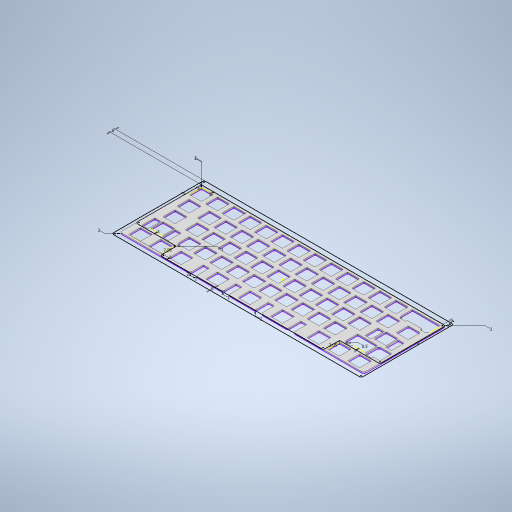
# Autodesk Inventor part: cast
Saved by Autodesk Inventor 2023 (Build 270158000, 158)
## iProperties
Created: 2023-09-13
Part Number: cast
Material: Generic
Document SubType Name: Modeling
Designer: Eric
Density: 1 g/cm^3
Appearance: Default
Author: Eric
Autodesk Inventor part; units mm, degrees
ref_plane "YZ Plane" through (0, 0, 0) normal (1, 0, 0) x (0, 1, 0)
ref_plane "XZ Plane" through (0, 0, 0) normal (0, 1, 0) x (-1, 0, 0)
ref_plane "XY Plane" through (0, 0, 0) normal (0, 0, 1) x (1, 0, 0)
sketch "Sketch1" plane through (0, 0, 0) normal (0, 1, 0) x (-1, 0, 0)
  line L0 (139.85, -45.1) -> (126.85, -45.1)
  line L1 (139.85, -31.1) -> (126.85, -31.1)
  line L2 (140.35, -44.6) -> (140.35, -31.6)
  line L3 (126.35, -44.6) -> (126.35, -31.6)
  arc A0 (139.85, -45.1) -> (140.35, -44.6) centre (139.85, -44.6) ccw
  arc A1 (126.35, -44.6) -> (126.85, -45.1) centre (126.85, -44.6) ccw
  arc A2 (140.35, -31.6) -> (139.85, -31.1) centre (139.85, -31.6) ccw
  arc A3 (126.85, -31.1) -> (126.35, -31.6) centre (126.85, -31.6) ccw
  line L4 (120.8, -45.1) -> (107.8, -45.1)
  line L5 (120.8, -31.1) -> (107.8, -31.1)
  line L6 (121.3, -44.6) -> (121.3, -31.6)
  line L7 (107.3, -44.6) -> (107.3, -31.6)
  arc A4 (120.8, -45.1) -> (121.3, -44.6) centre (120.8, -44.6) ccw
  arc A5 (107.3, -44.6) -> (107.8, -45.1) centre (107.8, -44.6) ccw
  arc A6 (121.3, -31.6) -> (120.8, -31.1) centre (120.8, -31.6) ccw
  arc A7 (107.8, -31.1) -> (107.3, -31.6) centre (107.8, -31.6) ccw
  line L8 (101.75, -45.1) -> (88.75, -45.1)
  line L9 (101.75, -31.1) -> (88.75, -31.1)
  line L10 (102.25, -44.6) -> (102.25, -31.6)
  line L11 (88.25, -44.6) -> (88.25, -31.6)
  arc A8 (101.75, -45.1) -> (102.25, -44.6) centre (101.75, -44.6) ccw
  arc A9 (88.25, -44.6) -> (88.75, -45.1) centre (88.75, -44.6) ccw
  arc A10 (102.25, -31.6) -> (101.75, -31.1) centre (101.75, -31.6) ccw
  arc A11 (88.75, -31.1) -> (88.25, -31.6) centre (88.75, -31.6) ccw
  line L12 (82.7, -45.1) -> (69.7, -45.1)
  line L13 (82.7, -31.1) -> (69.7, -31.1)
  line L14 (83.2, -44.6) -> (83.2, -31.6)
  line L15 (69.2, -44.6) -> (69.2, -31.6)
  arc A12 (82.7, -45.1) -> (83.2, -44.6) centre (82.7, -44.6) ccw
  arc A13 (69.2, -44.6) -> (69.7, -45.1) centre (69.7, -44.6) ccw
  arc A14 (83.2, -31.6) -> (82.7, -31.1) centre (82.7, -31.6) ccw
  arc A15 (69.7, -31.1) -> (69.2, -31.6) centre (69.7, -31.6) ccw
  line L16 (63.65, -45.1) -> (50.65, -45.1)
  line L17 (63.65, -31.1) -> (50.65, -31.1)
  line L18 (64.15, -44.6) -> (64.15, -31.6)
  line L19 (50.15, -44.6) -> (50.15, -31.6)
  arc A16 (63.65, -45.1) -> (64.15, -44.6) centre (63.65, -44.6) ccw
  arc A17 (50.15, -44.6) -> (50.65, -45.1) centre (50.65, -44.6) ccw
  arc A18 (64.15, -31.6) -> (63.65, -31.1) centre (63.65, -31.6) ccw
  arc A19 (50.65, -31.1) -> (50.15, -31.6) centre (50.65, -31.6) ccw
  line L20 (44.6, -45.1) -> (31.6, -45.1)
  line L21 (44.6, -31.1) -> (31.6, -31.1)
  line L22 (45.1, -44.6) -> (45.1, -31.6)
  line L23 (31.1, -44.6) -> (31.1, -31.6)
  arc A20 (44.6, -45.1) -> (45.1, -44.6) centre (44.6, -44.6) ccw
  arc A21 (31.1, -44.6) -> (31.6, -45.1) centre (31.6, -44.6) ccw
  arc A22 (45.1, -31.6) -> (44.6, -31.1) centre (44.6, -31.6) ccw
  arc A23 (31.6, -31.1) -> (31.1, -31.6) centre (31.6, -31.6) ccw
  line L24 (25.55, -45.1) -> (12.55, -45.1)
  line L25 (25.55, -31.1) -> (12.55, -31.1)
  line L26 (26.05, -44.6) -> (26.05, -31.6)
  line L27 (12.05, -44.6) -> (12.05, -31.6)
  arc A24 (25.55, -45.1) -> (26.05, -44.6) centre (25.55, -44.6) ccw
  arc A25 (12.05, -44.6) -> (12.55, -45.1) centre (12.55, -44.6) ccw
  arc A26 (26.05, -31.6) -> (25.55, -31.1) centre (25.55, -31.6) ccw
  arc A27 (12.55, -31.1) -> (12.05, -31.6) centre (12.55, -31.6) ccw
  line L28 (6.5, -45.1) -> (-6.5, -45.1)
  line L29 (6.5, -31.1) -> (-6.5, -31.1)
  line L30 (7, -44.6) -> (7, -31.6)
  line L31 (-7, -44.6) -> (-7, -31.6)
  arc A28 (6.5, -45.1) -> (7, -44.6) centre (6.5, -44.6) ccw
  arc A29 (-7, -44.6) -> (-6.5, -45.1) centre (-6.5, -44.6) ccw
  arc A30 (7, -31.6) -> (6.5, -31.1) centre (6.5, -31.6) ccw
  arc A31 (-6.5, -31.1) -> (-7, -31.6) centre (-6.5, -31.6) ccw
  line L32 (-12.55, -45.1) -> (-25.55, -45.1)
  line L33 (-12.55, -31.1) -> (-25.55, -31.1)
  line L34 (-12.05, -44.6) -> (-12.05, -31.6)
  line L35 (-26.05, -44.6) -> (-26.05, -31.6)
  arc A32 (-12.55, -45.1) -> (-12.05, -44.6) centre (-12.55, -44.6) ccw
  arc A33 (-26.05, -44.6) -> (-25.55, -45.1) centre (-25.55, -44.6) ccw
  arc A34 (-12.05, -31.6) -> (-12.55, -31.1) centre (-12.55, -31.6) ccw
  arc A35 (-25.55, -31.1) -> (-26.05, -31.6) centre (-25.55, -31.6) ccw
  line L36 (-31.6, -45.1) -> (-44.6, -45.1)
  line L37 (-31.6, -31.1) -> (-44.6, -31.1)
  line L38 (-31.1, -44.6) -> (-31.1, -31.6)
  line L39 (-45.1, -44.6) -> (-45.1, -31.6)
  arc A36 (-31.6, -45.1) -> (-31.1, -44.6) centre (-31.6, -44.6) ccw
  arc A37 (-45.1, -44.6) -> (-44.6, -45.1) centre (-44.6, -44.6) ccw
  arc A38 (-31.1, -31.6) -> (-31.6, -31.1) centre (-31.6, -31.6) ccw
  arc A39 (-44.6, -31.1) -> (-45.1, -31.6) centre (-44.6, -31.6) ccw
  line L40 (-50.65, -45.1) -> (-63.65, -45.1)
  line L41 (-50.65, -31.1) -> (-63.65, -31.1)
  line L42 (-50.15, -44.6) -> (-50.15, -31.6)
  line L43 (-64.15, -44.6) -> (-64.15, -31.6)
  arc A40 (-50.65, -45.1) -> (-50.15, -44.6) centre (-50.65, -44.6) ccw
  arc A41 (-64.15, -44.6) -> (-63.65, -45.1) centre (-63.65, -44.6) ccw
  arc A42 (-50.15, -31.6) -> (-50.65, -31.1) centre (-50.65, -31.6) ccw
  arc A43 (-63.65, -31.1) -> (-64.15, -31.6) centre (-63.65, -31.6) ccw
  line L44 (-69.7, -45.1) -> (-82.7, -45.1)
  line L45 (-69.7, -31.1) -> (-82.7, -31.1)
  line L46 (-69.2, -44.6) -> (-69.2, -31.6)
  line L47 (-83.2, -44.6) -> (-83.2, -31.6)
  arc A44 (-69.7, -45.1) -> (-69.2, -44.6) centre (-69.7, -44.6) ccw
  arc A45 (-83.2, -44.6) -> (-82.7, -45.1) centre (-82.7, -44.6) ccw
  arc A46 (-69.2, -31.6) -> (-69.7, -31.1) centre (-69.7, -31.6) ccw
  arc A47 (-82.7, -31.1) -> (-83.2, -31.6) centre (-82.7, -31.6) ccw
  line L48 (-88.75, -45.1) -> (-101.75, -45.1)
  line L49 (-88.75, -31.1) -> (-101.75, -31.1)
  line L50 (-88.25, -44.6) -> (-88.25, -31.6)
  line L51 (-102.25, -44.6) -> (-102.25, -31.6)
  arc A48 (-88.75, -45.1) -> (-88.25, -44.6) centre (-88.75, -44.6) ccw
  arc A49 (-102.25, -44.6) -> (-101.75, -45.1) centre (-101.75, -44.6) ccw
  arc A50 (-88.25, -31.6) -> (-88.75, -31.1) centre (-88.75, -31.6) ccw
  arc A51 (-101.75, -31.1) -> (-102.25, -31.6) centre (-101.75, -31.6) ccw
  line L52 (-107.8, -45.1) -> (-120.8, -45.1)
  line L53 (-107.3, -44.6) -> (-107.3, -31.6)
  arc A52 (-107.8, -45.1) -> (-107.3, -44.6) centre (-107.8, -44.6) ccw
  arc A53 (-107.3, -31.6) -> (-107.8, -31.1) centre (-107.8, -31.6) ccw
  line L54 (-117.325, -45.1) -> (-130.325, -45.1)
  line L55 (-117.325, -31.1) -> (-130.325, -31.1)
  line L56 (-108.887, -29.1) -> (-114.887, -29.1)
  line L57 (-108.387, -30.6) -> (-108.387, -29.6)
  line L58 (-115.387, -30.6) -> (-115.387, -29.6)
  arc A54 (-108.387, -29.6) -> (-108.887, -29.1) centre (-108.887, -29.6) ccw
  arc A55 (-114.887, -29.1) -> (-115.387, -29.6) centre (-114.887, -29.6) ccw
  line L59 (-132.763, -29.1) -> (-138.763, -29.1)
  line L60 (-132.263, -30.6) -> (-132.263, -29.6)
  line L61 (-139.263, -30.6) -> (-139.263, -29.6)
  arc A56 (-132.263, -29.6) -> (-132.763, -29.1) centre (-132.763, -29.6) ccw
  arc A57 (-138.763, -29.1) -> (-139.263, -29.6) centre (-138.763, -29.6) ccw
  line L62 (-126.85, -45.1) -> (-139.85, -45.1)
  line L63 (-140.35, -44.6) -> (-140.35, -31.6)
  arc A58 (-140.35, -44.6) -> (-139.85, -45.1) centre (-139.85, -44.6) ccw
  arc A59 (-139.85, -31.1) -> (-140.35, -31.6) centre (-139.85, -31.6) ccw
  line L64 (135.0875, -26.05) -> (122.0875, -26.05)
  line L65 (135.0875, -12.05) -> (122.0875, -12.05)
  line L66 (135.5875, -25.55) -> (135.5875, -12.55)
  line L67 (121.5875, -25.55) -> (121.5875, -12.55)
  arc A60 (135.0875, -26.05) -> (135.5875, -25.55) centre (135.0875, -25.55) ccw
  arc A61 (121.5875, -25.55) -> (122.0875, -26.05) centre (122.0875, -25.55) ccw
  arc A62 (135.5875, -12.55) -> (135.0875, -12.05) centre (135.0875, -12.55) ccw
  arc A63 (122.0875, -12.05) -> (121.5875, -12.55) centre (122.0875, -12.55) ccw
  line L68 (111.275, -26.05) -> (98.275, -26.05)
  line L69 (111.275, -12.05) -> (98.275, -12.05)
  line L70 (111.775, -25.55) -> (111.775, -12.55)
  line L71 (97.775, -25.55) -> (97.775, -12.55)
  arc A64 (111.275, -26.05) -> (111.775, -25.55) centre (111.275, -25.55) ccw
  arc A65 (97.775, -25.55) -> (98.275, -26.05) centre (98.275, -25.55) ccw
  arc A66 (111.775, -12.55) -> (111.275, -12.05) centre (111.275, -12.55) ccw
  arc A67 (98.275, -12.05) -> (97.775, -12.55) centre (98.275, -12.55) ccw
  line L72 (92.225, -26.05) -> (79.225, -26.05)
  line L73 (92.225, -12.05) -> (79.225, -12.05)
  line L74 (92.725, -25.55) -> (92.725, -12.55)
  line L75 (78.725, -25.55) -> (78.725, -12.55)
  arc A68 (92.225, -26.05) -> (92.725, -25.55) centre (92.225, -25.55) ccw
  arc A69 (78.725, -25.55) -> (79.225, -26.05) centre (79.225, -25.55) ccw
  arc A70 (92.725, -12.55) -> (92.225, -12.05) centre (92.225, -12.55) ccw
  arc A71 (79.225, -12.05) -> (78.725, -12.55) centre (79.225, -12.55) ccw
  line L76 (73.175, -26.05) -> (60.175, -26.05)
  line L77 (73.175, -12.05) -> (60.175, -12.05)
  line L78 (73.675, -25.55) -> (73.675, -12.55)
  line L79 (59.675, -25.55) -> (59.675, -12.55)
  arc A72 (73.175, -26.05) -> (73.675, -25.55) centre (73.175, -25.55) ccw
  arc A73 (59.675, -25.55) -> (60.175, -26.05) centre (60.175, -25.55) ccw
  arc A74 (73.675, -12.55) -> (73.175, -12.05) centre (73.175, -12.55) ccw
  arc A75 (60.175, -12.05) -> (59.675, -12.55) centre (60.175, -12.55) ccw
  line L80 (54.125, -26.05) -> (41.125, -26.05)
  line L81 (54.125, -12.05) -> (41.125, -12.05)
  line L82 (54.625, -25.55) -> (54.625, -12.55)
  line L83 (40.625, -25.55) -> (40.625, -12.55)
  arc A76 (54.125, -26.05) -> (54.625, -25.55) centre (54.125, -25.55) ccw
  arc A77 (40.625, -25.55) -> (41.125, -26.05) centre (41.125, -25.55) ccw
  arc A78 (54.625, -12.55) -> (54.125, -12.05) centre (54.125, -12.55) ccw
  arc A79 (41.125, -12.05) -> (40.625, -12.55) centre (41.125, -12.55) ccw
  line L84 (35.075, -26.05) -> (22.075, -26.05)
  line L85 (35.075, -12.05) -> (22.075, -12.05)
  line L86 (35.575, -25.55) -> (35.575, -12.55)
  line L87 (21.575, -25.55) -> (21.575, -12.55)
  arc A80 (35.075, -26.05) -> (35.575, -25.55) centre (35.075, -25.55) ccw
  arc A81 (21.575, -25.55) -> (22.075, -26.05) centre (22.075, -25.55) ccw
  arc A82 (35.575, -12.55) -> (35.075, -12.05) centre (35.075, -12.55) ccw
  arc A83 (22.075, -12.05) -> (21.575, -12.55) centre (22.075, -12.55) ccw
  line L88 (16.025, -26.05) -> (3.025, -26.05)
  line L89 (16.025, -12.05) -> (3.025, -12.05)
  line L90 (16.525, -25.55) -> (16.525, -12.55)
  line L91 (2.525, -25.55) -> (2.525, -12.55)
  arc A84 (16.025, -26.05) -> (16.525, -25.55) centre (16.025, -25.55) ccw
  arc A85 (2.525, -25.55) -> (3.025, -26.05) centre (3.025, -25.55) ccw
  arc A86 (16.525, -12.55) -> (16.025, -12.05) centre (16.025, -12.55) ccw
  arc A87 (3.025, -12.05) -> (2.525, -12.55) centre (3.025, -12.55) ccw
  line L92 (-3.025, -26.05) -> (-16.025, -26.05)
  line L93 (-3.025, -12.05) -> (-16.025, -12.05)
  line L94 (-2.525, -25.55) -> (-2.525, -12.55)
  line L95 (-16.525, -25.55) -> (-16.525, -12.55)
  arc A88 (-3.025, -26.05) -> (-2.525, -25.55) centre (-3.025, -25.55) ccw
  arc A89 (-16.525, -25.55) -> (-16.025, -26.05) centre (-16.025, -25.55) ccw
  arc A90 (-2.525, -12.55) -> (-3.025, -12.05) centre (-3.025, -12.55) ccw
  arc A91 (-16.025, -12.05) -> (-16.525, -12.55) centre (-16.025, -12.55) ccw
  line L96 (-22.075, -26.05) -> (-35.075, -26.05)
  line L97 (-22.075, -12.05) -> (-35.075, -12.05)
  line L98 (-21.575, -25.55) -> (-21.575, -12.55)
  line L99 (-35.575, -25.55) -> (-35.575, -12.55)
  arc A92 (-22.075, -26.05) -> (-21.575, -25.55) centre (-22.075, -25.55) ccw
  arc A93 (-35.575, -25.55) -> (-35.075, -26.05) centre (-35.075, -25.55) ccw
  arc A94 (-21.575, -12.55) -> (-22.075, -12.05) centre (-22.075, -12.55) ccw
  arc A95 (-35.075, -12.05) -> (-35.575, -12.55) centre (-35.075, -12.55) ccw
  line L100 (-41.125, -26.05) -> (-54.125, -26.05)
  line L101 (-41.125, -12.05) -> (-54.125, -12.05)
  line L102 (-40.625, -25.55) -> (-40.625, -12.55)
  line L103 (-54.625, -25.55) -> (-54.625, -12.55)
  arc A96 (-41.125, -26.05) -> (-40.625, -25.55) centre (-41.125, -25.55) ccw
  arc A97 (-54.625, -25.55) -> (-54.125, -26.05) centre (-54.125, -25.55) ccw
  arc A98 (-40.625, -12.55) -> (-41.125, -12.05) centre (-41.125, -12.55) ccw
  arc A99 (-54.125, -12.05) -> (-54.625, -12.55) centre (-54.125, -12.55) ccw
  line L104 (-60.175, -26.05) -> (-73.175, -26.05)
  line L105 (-60.175, -12.05) -> (-73.175, -12.05)
  line L106 (-59.675, -25.55) -> (-59.675, -12.55)
  line L107 (-73.675, -25.55) -> (-73.675, -12.55)
  arc A100 (-60.175, -26.05) -> (-59.675, -25.55) centre (-60.175, -25.55) ccw
  arc A101 (-73.675, -25.55) -> (-73.175, -26.05) centre (-73.175, -25.55) ccw
  arc A102 (-59.675, -12.55) -> (-60.175, -12.05) centre (-60.175, -12.55) ccw
  arc A103 (-73.175, -12.05) -> (-73.675, -12.55) centre (-73.175, -12.55) ccw
  line L108 (-79.225, -26.05) -> (-92.225, -26.05)
  line L109 (-79.225, -12.05) -> (-92.225, -12.05)
  line L110 (-78.725, -25.55) -> (-78.725, -12.55)
  line L111 (-92.725, -25.55) -> (-92.725, -12.55)
  arc A104 (-79.225, -26.05) -> (-78.725, -25.55) centre (-79.225, -25.55) ccw
  arc A105 (-92.725, -25.55) -> (-92.225, -26.05) centre (-92.225, -25.55) ccw
  arc A106 (-78.725, -12.55) -> (-79.225, -12.05) centre (-79.225, -12.55) ccw
  arc A107 (-92.225, -12.05) -> (-92.725, -12.55) centre (-92.225, -12.55) ccw
  line L112 (-98.275, -26.05) -> (-111.275, -26.05)
  line L113 (-98.275, -12.05) -> (-111.275, -12.05)
  line L114 (-97.775, -25.55) -> (-97.775, -12.55)
  line L115 (-111.775, -25.55) -> (-111.775, -12.55)
  arc A108 (-98.275, -26.05) -> (-97.775, -25.55) centre (-98.275, -25.55) ccw
  arc A109 (-111.775, -25.55) -> (-111.275, -26.05) centre (-111.275, -25.55) ccw
  arc A110 (-97.775, -12.55) -> (-98.275, -12.05) centre (-98.275, -12.55) ccw
  arc A111 (-111.275, -12.05) -> (-111.775, -12.55) centre (-111.275, -12.55) ccw
  line L116 (-122.0875, -26.05) -> (-135.0875, -26.05)
  line L117 (-122.0875, -12.05) -> (-135.0875, -12.05)
  line L118 (-121.5875, -25.55) -> (-121.5875, -12.55)
  line L119 (-135.5875, -25.55) -> (-135.5875, -12.55)
  arc A112 (-122.0875, -26.05) -> (-121.5875, -25.55) centre (-122.0875, -25.55) ccw
  arc A113 (-135.5875, -25.55) -> (-135.0875, -26.05) centre (-135.0875, -25.55) ccw
  arc A114 (-121.5875, -12.55) -> (-122.0875, -12.05) centre (-122.0875, -12.55) ccw
  arc A115 (-135.0875, -12.05) -> (-135.5875, -12.55) centre (-135.0875, -12.55) ccw
  line L120 (132.7062, -7) -> (119.7062, -7)
  line L121 (132.7062, 7) -> (119.7062, 7)
  line L122 (133.2063, -6.5) -> (133.2063, 6.5)
  line L123 (119.2062, -6.5) -> (119.2062, 6.5)
  arc A116 (132.7062, -7) -> (133.2063, -6.5) centre (132.7062, -6.5) ccw
  arc A117 (119.2062, -6.5) -> (119.7062, -7) centre (119.7062, -6.5) ccw
  arc A118 (133.2063, 6.5) -> (132.7062, 7) centre (132.7062, 6.5) ccw
  arc A119 (119.7062, 7) -> (119.2062, 6.5) centre (119.7062, 6.5) ccw
  line L124 (106.5125, -7) -> (93.5125, -7)
  line L125 (106.5125, 7) -> (93.5125, 7)
  line L126 (107.0125, -6.5) -> (107.0125, 6.5)
  line L127 (93.0125, -6.5) -> (93.0125, 6.5)
  arc A120 (106.5125, -7) -> (107.0125, -6.5) centre (106.5125, -6.5) ccw
  arc A121 (93.0125, -6.5) -> (93.5125, -7) centre (93.5125, -6.5) ccw
  arc A122 (107.0125, 6.5) -> (106.5125, 7) centre (106.5125, 6.5) ccw
  arc A123 (93.5125, 7) -> (93.0125, 6.5) centre (93.5125, 6.5) ccw
  line L128 (87.4625, -7) -> (74.4625, -7)
  line L129 (87.4625, 7) -> (74.4625, 7)
  line L130 (87.9625, -6.5) -> (87.9625, 6.5)
  line L131 (73.9625, -6.5) -> (73.9625, 6.5)
  arc A124 (87.4625, -7) -> (87.9625, -6.5) centre (87.4625, -6.5) ccw
  arc A125 (73.9625, -6.5) -> (74.4625, -7) centre (74.4625, -6.5) ccw
  arc A126 (87.9625, 6.5) -> (87.4625, 7) centre (87.4625, 6.5) ccw
  arc A127 (74.4625, 7) -> (73.9625, 6.5) centre (74.4625, 6.5) ccw
  line L132 (68.4125, -7) -> (55.4125, -7)
  line L133 (68.4125, 7) -> (55.4125, 7)
  line L134 (68.9125, -6.5) -> (68.9125, 6.5)
  line L135 (54.9125, -6.5) -> (54.9125, 6.5)
  arc A128 (68.4125, -7) -> (68.9125, -6.5) centre (68.4125, -6.5) ccw
  arc A129 (54.9125, -6.5) -> (55.4125, -7) centre (55.4125, -6.5) ccw
  arc A130 (68.9125, 6.5) -> (68.4125, 7) centre (68.4125, 6.5) ccw
  arc A131 (55.4125, 7) -> (54.9125, 6.5) centre (55.4125, 6.5) ccw
  line L136 (49.3625, -7) -> (36.3625, -7)
  line L137 (49.3625, 7) -> (36.3625, 7)
  line L138 (49.8625, -6.5) -> (49.8625, 6.5)
  line L139 (35.8625, -6.5) -> (35.8625, 6.5)
  arc A132 (49.3625, -7) -> (49.8625, -6.5) centre (49.3625, -6.5) ccw
  arc A133 (35.8625, -6.5) -> (36.3625, -7) centre (36.3625, -6.5) ccw
  arc A134 (49.8625, 6.5) -> (49.3625, 7) centre (49.3625, 6.5) ccw
  arc A135 (36.3625, 7) -> (35.8625, 6.5) centre (36.3625, 6.5) ccw
  line L140 (30.3125, -7) -> (17.3125, -7)
  line L141 (30.3125, 7) -> (17.3125, 7)
  line L142 (30.8125, -6.5) -> (30.8125, 6.5)
  line L143 (16.8125, -6.5) -> (16.8125, 6.5)
  arc A136 (30.3125, -7) -> (30.8125, -6.5) centre (30.3125, -6.5) ccw
  arc A137 (16.8125, -6.5) -> (17.3125, -7) centre (17.3125, -6.5) ccw
  arc A138 (30.8125, 6.5) -> (30.3125, 7) centre (30.3125, 6.5) ccw
  arc A139 (17.3125, 7) -> (16.8125, 6.5) centre (17.3125, 6.5) ccw
  line L144 (11.2625, -7) -> (-1.7375, -7)
  line L145 (11.2625, 7) -> (-1.7375, 7)
  line L146 (11.7625, -6.5) -> (11.7625, 6.5)
  line L147 (-2.2375, -6.5) -> (-2.2375, 6.5)
  arc A140 (11.2625, -7) -> (11.7625, -6.5) centre (11.2625, -6.5) ccw
  arc A141 (-2.2375, -6.5) -> (-1.7375, -7) centre (-1.7375, -6.5) ccw
  arc A142 (11.7625, 6.5) -> (11.2625, 7) centre (11.2625, 6.5) ccw
  arc A143 (-1.7375, 7) -> (-2.2375, 6.5) centre (-1.7375, 6.5) ccw
  line L148 (-7.7875, -7) -> (-20.7875, -7)
  line L149 (-7.7875, 7) -> (-20.7875, 7)
  line L150 (-7.2875, -6.5) -> (-7.2875, 6.5)
  line L151 (-21.2875, -6.5) -> (-21.2875, 6.5)
  arc A144 (-7.7875, -7) -> (-7.2875, -6.5) centre (-7.7875, -6.5) ccw
  arc A145 (-21.2875, -6.5) -> (-20.7875, -7) centre (-20.7875, -6.5) ccw
  arc A146 (-7.2875, 6.5) -> (-7.7875, 7) centre (-7.7875, 6.5) ccw
  arc A147 (-20.7875, 7) -> (-21.2875, 6.5) centre (-20.7875, 6.5) ccw
  line L152 (-26.8375, -7) -> (-39.8375, -7)
  line L153 (-26.8375, 7) -> (-39.8375, 7)
  line L154 (-26.3375, -6.5) -> (-26.3375, 6.5)
  line L155 (-40.3375, -6.5) -> (-40.3375, 6.5)
  arc A148 (-26.8375, -7) -> (-26.3375, -6.5) centre (-26.8375, -6.5) ccw
  arc A149 (-40.3375, -6.5) -> (-39.8375, -7) centre (-39.8375, -6.5) ccw
  arc A150 (-26.3375, 6.5) -> (-26.8375, 7) centre (-26.8375, 6.5) ccw
  arc A151 (-39.8375, 7) -> (-40.3375, 6.5) centre (-39.8375, 6.5) ccw
  line L156 (-45.8875, -7) -> (-58.8875, -7)
  line L157 (-45.8875, 7) -> (-58.8875, 7)
  line L158 (-45.3875, -6.5) -> (-45.3875, 6.5)
  line L159 (-59.3875, -6.5) -> (-59.3875, 6.5)
  arc A152 (-45.8875, -7) -> (-45.3875, -6.5) centre (-45.8875, -6.5) ccw
  arc A153 (-59.3875, -6.5) -> (-58.8875, -7) centre (-58.8875, -6.5) ccw
  arc A154 (-45.3875, 6.5) -> (-45.8875, 7) centre (-45.8875, 6.5) ccw
  arc A155 (-58.8875, 7) -> (-59.3875, 6.5) centre (-58.8875, 6.5) ccw
  line L160 (-64.9375, -7) -> (-77.9375, -7)
  line L161 (-64.9375, 7) -> (-77.9375, 7)
  line L162 (-64.4375, -6.5) -> (-64.4375, 6.5)
  line L163 (-78.4375, -6.5) -> (-78.4375, 6.5)
  arc A156 (-64.9375, -7) -> (-64.4375, -6.5) centre (-64.9375, -6.5) ccw
  arc A157 (-78.4375, -6.5) -> (-77.9375, -7) centre (-77.9375, -6.5) ccw
  arc A158 (-64.4375, 6.5) -> (-64.9375, 7) centre (-64.9375, 6.5) ccw
  arc A159 (-77.9375, 7) -> (-78.4375, 6.5) centre (-77.9375, 6.5) ccw
  line L164 (-83.9875, -7) -> (-96.9875, -7)
  line L165 (-83.9875, 7) -> (-96.9875, 7)
  line L166 (-83.4875, -6.5) -> (-83.4875, 6.5)
  line L167 (-97.4875, -6.5) -> (-97.4875, 6.5)
  arc A160 (-83.9875, -7) -> (-83.4875, -6.5) centre (-83.9875, -6.5) ccw
  arc A161 (-97.4875, -6.5) -> (-96.9875, -7) centre (-96.9875, -6.5) ccw
  arc A162 (-83.4875, 6.5) -> (-83.9875, 7) centre (-83.9875, 6.5) ccw
  arc A163 (-96.9875, 7) -> (-97.4875, 6.5) centre (-96.9875, 6.5) ccw
  line L168 (-114.9437, -7) -> (-127.9437, -7)
  line L169 (-114.9437, 7) -> (-127.9437, 7)
  line L170 (-114.4438, -6.5) -> (-114.4437, 6.5)
  line L171 (-128.4438, -6.5) -> (-128.4437, 6.5)
  arc A164 (-114.9437, -7) -> (-114.4438, -6.5) centre (-114.9438, -6.5) ccw
  arc A165 (-128.4438, -6.5) -> (-127.9437, -7) centre (-127.9437, -6.5) ccw
  arc A166 (-114.4437, 6.5) -> (-114.9437, 7) centre (-114.9437, 6.5) ccw
  arc A167 (-127.9437, 7) -> (-128.4437, 6.5) centre (-127.9437, 6.5) ccw
  line L172 (-106.5058, -6) -> (-112.5057, -6)
  line L173 (-106.5057, 9) -> (-112.5057, 9)
  line L174 (-106.0057, -5.5) -> (-106.0057, 8.5)
  line L175 (-113.0058, -5.5) -> (-113.0058, 8.5)
  arc A168 (-106.5058, -6) -> (-106.0057, -5.5) centre (-106.5057, -5.5) ccw
  arc A169 (-113.0058, -5.5) -> (-112.5057, -6) centre (-112.5058, -5.5) ccw
  arc A170 (-106.0057, 8.5) -> (-106.5057, 9) centre (-106.5057, 8.5) ccw
  arc A171 (-112.5057, 9) -> (-113.0058, 8.5) centre (-112.5058, 8.5) ccw
  line L176 (-130.3818, -6) -> (-136.3818, -6)
  line L177 (-130.3817, 9) -> (-136.3818, 9)
  line L178 (-129.8818, -5.5) -> (-129.8818, 8.5)
  line L179 (-136.8817, -5.5) -> (-136.8817, 8.5)
  arc A172 (-130.3818, -6) -> (-129.8818, -5.5) centre (-130.3818, -5.5) ccw
  arc A173 (-136.8817, -5.5) -> (-136.3818, -6) centre (-136.3817, -5.5) ccw
  arc A174 (-129.8818, 8.5) -> (-130.3817, 9) centre (-130.3818, 8.5) ccw
  arc A175 (-136.3818, 9) -> (-136.8817, 8.5) centre (-136.3818, 8.5) ccw
  line L180 (127.9437, 12.05) -> (114.9438, 12.05)
  line L181 (127.9437, 26.05) -> (114.9437, 26.05)
  line L182 (128.4437, 12.55) -> (128.4437, 25.55)
  line L183 (114.4437, 12.55) -> (114.4437, 25.55)
  arc A176 (127.9437, 12.05) -> (128.4437, 12.55) centre (127.9437, 12.55) ccw
  arc A177 (114.4437, 12.55) -> (114.9438, 12.05) centre (114.9437, 12.55) ccw
  arc A178 (128.4437, 25.55) -> (127.9437, 26.05) centre (127.9437, 25.55) ccw
  arc A179 (114.9437, 26.05) -> (114.4437, 25.55) centre (114.9437, 25.55) ccw
  line L184 (136.3818, 13.05) -> (130.3817, 13.05)
  line L185 (136.3817, 28.05) -> (130.3817, 28.05)
  line L186 (136.8817, 13.55) -> (136.8817, 27.55)
  line L187 (129.8817, 13.55) -> (129.8817, 27.55)
  arc A180 (136.3818, 13.05) -> (136.8817, 13.55) centre (136.3817, 13.55) ccw
  arc A181 (129.8817, 13.55) -> (130.3817, 13.05) centre (130.3817, 13.55) ccw
  arc A182 (136.8817, 27.55) -> (136.3817, 28.05) centre (136.3817, 27.55) ccw
  arc A183 (130.3817, 28.05) -> (129.8817, 27.55) centre (130.3817, 27.55) ccw
  line L188 (112.5057, 13.05) -> (106.5058, 13.05)
  line L189 (112.5057, 28.05) -> (106.5057, 28.05)
  line L190 (113.0057, 13.55) -> (113.0058, 27.55)
  line L191 (106.0057, 13.55) -> (106.0057, 27.55)
  arc A184 (112.5057, 13.05) -> (113.0057, 13.55) centre (112.5057, 13.55) ccw
  arc A185 (106.0057, 13.55) -> (106.5058, 13.05) centre (106.5057, 13.55) ccw
  arc A186 (113.0058, 27.55) -> (112.5057, 28.05) centre (112.5058, 27.55) ccw
  arc A187 (106.5057, 28.05) -> (106.0057, 27.55) centre (106.5058, 27.55) ccw
  line L192 (96.9875, 12.05) -> (83.9875, 12.05)
  line L193 (96.9875, 26.05) -> (83.9875, 26.05)
  line L194 (97.4875, 12.55) -> (97.4875, 25.55)
  line L195 (83.4875, 12.55) -> (83.4875, 25.55)
  arc A188 (96.9875, 12.05) -> (97.4875, 12.55) centre (96.9875, 12.55) ccw
  arc A189 (83.4875, 12.55) -> (83.9875, 12.05) centre (83.9875, 12.55) ccw
  arc A190 (97.4875, 25.55) -> (96.9875, 26.05) centre (96.9875, 25.55) ccw
  arc A191 (83.9875, 26.05) -> (83.4875, 25.55) centre (83.9875, 25.55) ccw
  line L196 (77.9375, 12.05) -> (64.9375, 12.05)
  line L197 (77.9375, 26.05) -> (64.9375, 26.05)
  line L198 (78.4375, 12.55) -> (78.4375, 25.55)
  line L199 (64.4375, 12.55) -> (64.4375, 25.55)
  arc A192 (77.9375, 12.05) -> (78.4375, 12.55) centre (77.9375, 12.55) ccw
  arc A193 (64.4375, 12.55) -> (64.9375, 12.05) centre (64.9375, 12.55) ccw
  arc A194 (78.4375, 25.55) -> (77.9375, 26.05) centre (77.9375, 25.55) ccw
  arc A195 (64.9375, 26.05) -> (64.4375, 25.55) centre (64.9375, 25.55) ccw
  line L200 (58.8875, 12.05) -> (45.8875, 12.05)
  line L201 (58.8875, 26.05) -> (45.8875, 26.05)
  line L202 (59.3875, 12.55) -> (59.3875, 25.55)
  line L203 (45.3875, 12.55) -> (45.3875, 25.55)
  arc A196 (58.8875, 12.05) -> (59.3875, 12.55) centre (58.8875, 12.55) ccw
  arc A197 (45.3875, 12.55) -> (45.8875, 12.05) centre (45.8875, 12.55) ccw
  arc A198 (59.3875, 25.55) -> (58.8875, 26.05) centre (58.8875, 25.55) ccw
  arc A199 (45.8875, 26.05) -> (45.3875, 25.55) centre (45.8875, 25.55) ccw
  line L204 (39.8375, 12.05) -> (26.8375, 12.05)
  line L205 (39.8375, 26.05) -> (26.8375, 26.05)
  line L206 (40.3375, 12.55) -> (40.3375, 25.55)
  line L207 (26.3375, 12.55) -> (26.3375, 25.55)
  arc A200 (39.8375, 12.05) -> (40.3375, 12.55) centre (39.8375, 12.55) ccw
  arc A201 (26.3375, 12.55) -> (26.8375, 12.05) centre (26.8375, 12.55) ccw
  arc A202 (40.3375, 25.55) -> (39.8375, 26.05) centre (39.8375, 25.55) ccw
  arc A203 (26.8375, 26.05) -> (26.3375, 25.55) centre (26.8375, 25.55) ccw
  line L208 (20.7875, 12.05) -> (7.7875, 12.05)
  line L209 (20.7875, 26.05) -> (7.7875, 26.05)
  line L210 (21.2875, 12.55) -> (21.2875, 25.55)
  line L211 (7.2875, 12.55) -> (7.2875, 25.55)
  arc A204 (20.7875, 12.05) -> (21.2875, 12.55) centre (20.7875, 12.55) ccw
  arc A205 (7.2875, 12.55) -> (7.7875, 12.05) centre (7.7875, 12.55) ccw
  arc A206 (21.2875, 25.55) -> (20.7875, 26.05) centre (20.7875, 25.55) ccw
  arc A207 (7.7875, 26.05) -> (7.2875, 25.55) centre (7.7875, 25.55) ccw
  line L212 (1.7375, 12.05) -> (-11.2625, 12.05)
  line L213 (1.7375, 26.05) -> (-11.2625, 26.05)
  line L214 (2.2375, 12.55) -> (2.2375, 25.55)
  line L215 (-11.7625, 12.55) -> (-11.7625, 25.55)
  arc A208 (1.7375, 12.05) -> (2.2375, 12.55) centre (1.7375, 12.55) ccw
  arc A209 (-11.7625, 12.55) -> (-11.2625, 12.05) centre (-11.2625, 12.55) ccw
  arc A210 (2.2375, 25.55) -> (1.7375, 26.05) centre (1.7375, 25.55) ccw
  arc A211 (-11.2625, 26.05) -> (-11.7625, 25.55) centre (-11.2625, 25.55) ccw
  line L216 (-17.3125, 12.05) -> (-30.3125, 12.05)
  line L217 (-17.3125, 26.05) -> (-30.3125, 26.05)
  line L218 (-16.8125, 12.55) -> (-16.8125, 25.55)
  line L219 (-30.8125, 12.55) -> (-30.8125, 25.55)
  arc A212 (-17.3125, 12.05) -> (-16.8125, 12.55) centre (-17.3125, 12.55) ccw
  arc A213 (-30.8125, 12.55) -> (-30.3125, 12.05) centre (-30.3125, 12.55) ccw
  arc A214 (-16.8125, 25.55) -> (-17.3125, 26.05) centre (-17.3125, 25.55) ccw
  arc A215 (-30.3125, 26.05) -> (-30.8125, 25.55) centre (-30.3125, 25.55) ccw
  line L220 (-36.3625, 12.05) -> (-49.3625, 12.05)
  line L221 (-36.3625, 26.05) -> (-49.3625, 26.05)
  line L222 (-35.8625, 12.55) -> (-35.8625, 25.55)
  line L223 (-49.8625, 12.55) -> (-49.8625, 25.55)
  arc A216 (-36.3625, 12.05) -> (-35.8625, 12.55) centre (-36.3625, 12.55) ccw
  arc A217 (-49.8625, 12.55) -> (-49.3625, 12.05) centre (-49.3625, 12.55) ccw
  arc A218 (-35.8625, 25.55) -> (-36.3625, 26.05) centre (-36.3625, 25.55) ccw
  arc A219 (-49.3625, 26.05) -> (-49.8625, 25.55) centre (-49.3625, 25.55) ccw
  line L224 (-55.4125, 12.05) -> (-68.4125, 12.05)
  line L225 (-55.4125, 26.05) -> (-68.4125, 26.05)
  line L226 (-54.9125, 12.55) -> (-54.9125, 25.55)
  line L227 (-68.9125, 12.55) -> (-68.9125, 25.55)
  arc A220 (-55.4125, 12.05) -> (-54.9125, 12.55) centre (-55.4125, 12.55) ccw
  arc A221 (-68.9125, 12.55) -> (-68.4125, 12.05) centre (-68.4125, 12.55) ccw
  arc A222 (-54.9125, 25.55) -> (-55.4125, 26.05) centre (-55.4125, 25.55) ccw
  arc A223 (-68.4125, 26.05) -> (-68.9125, 25.55) centre (-68.4125, 25.55) ccw
  line L228 (-74.4625, 12.05) -> (-87.4625, 12.05)
  line L229 (-74.4625, 26.05) -> (-87.4625, 26.05)
  line L230 (-73.9625, 12.55) -> (-73.9625, 25.55)
  line L231 (-87.9625, 12.55) -> (-87.9625, 25.55)
  arc A224 (-74.4625, 12.05) -> (-73.9625, 12.55) centre (-74.4625, 12.55) ccw
  arc A225 (-87.9625, 12.55) -> (-87.4625, 12.05) centre (-87.4625, 12.55) ccw
  arc A226 (-73.9625, 25.55) -> (-74.4625, 26.05) centre (-74.4625, 25.55) ccw
  arc A227 (-87.4625, 26.05) -> (-87.9625, 25.55) centre (-87.4625, 25.55) ccw
  line L232 (-100.6562, 12.05) -> (-113.6563, 12.05)
  line L233 (-100.1562, 12.55) -> (-100.1563, 25.55)
  arc A228 (-100.6562, 12.05) -> (-100.1562, 12.55) centre (-100.6562, 12.55) ccw
  arc A229 (-100.1563, 25.55) -> (-100.6563, 26.05) centre (-100.6562, 25.55) ccw
  line L234 (-110.1812, 12.05) -> (-123.1812, 12.05)
  line L235 (-110.1812, 26.05) -> (-123.1813, 26.05)
  line L236 (-123.6812, 12.55) -> (-123.6812, 25.55)
  arc A230 (-123.6812, 12.55) -> (-123.1812, 12.05) centre (-123.1812, 12.55) ccw
  arc A231 (-123.1813, 26.05) -> (-123.6812, 25.55) centre (-123.1812, 25.55) ccw
  line L237 (-101.7432, 28.05) -> (-107.7432, 28.05)
  line L238 (-101.2432, 26.55) -> (-101.2432, 27.55)
  line L239 (-108.2433, 26.55) -> (-108.2433, 27.55)
  arc A232 (-101.2432, 27.55) -> (-101.7432, 28.05) centre (-101.7432, 27.55) ccw
  arc A233 (-107.7432, 28.05) -> (-108.2433, 27.55) centre (-107.7432, 27.55) ccw
  line L240 (-125.6193, 13.05) -> (-125.85, 13.05)
  line L241 (-125.6192, 28.05) -> (-131.6193, 28.05)
  line L242 (-125.1192, 13.55) -> (-125.1193, 27.55)
  line L243 (-132.1193, 26.55) -> (-132.1193, 27.55)
  arc A234 (-125.6193, 13.05) -> (-125.1192, 13.55) centre (-125.6192, 13.55) ccw
  arc A235 (-125.1193, 27.55) -> (-125.6192, 28.05) centre (-125.6193, 27.55) ccw
  arc A236 (-131.6193, 28.05) -> (-132.1193, 27.55) centre (-131.6193, 27.55) ccw
  line L244 (-126.85, 12.05) -> (-139.85, 12.05)
  line L245 (-132.6193, 26.05) -> (-139.85, 26.05)
  line L246 (-126.35, 12.55) -> (-126.35, 12.55)
  line L247 (-140.35, 12.55) -> (-140.35, 25.55)
  arc A237 (-126.85, 12.05) -> (-126.35, 12.55) centre (-126.85, 12.55) ccw
  arc A238 (-140.35, 12.55) -> (-139.85, 12.05) centre (-139.85, 12.55) ccw
  arc A239 (-139.85, 26.05) -> (-140.35, 25.55) centre (-139.85, 25.55) ccw
  line L248 (135.0875, 31.1) -> (122.0875, 31.1)
  line L249 (135.0875, 45.1) -> (122.0875, 45.1)
  line L250 (135.5875, 31.6) -> (135.5875, 44.6)
  line L251 (121.5875, 31.6) -> (121.5875, 44.6)
  arc A240 (135.0875, 31.1) -> (135.5875, 31.6) centre (135.0875, 31.6) ccw
  arc A241 (121.5875, 31.6) -> (122.0875, 31.1) centre (122.0875, 31.6) ccw
  arc A242 (135.5875, 44.6) -> (135.0875, 45.1) centre (135.0875, 44.6) ccw
  arc A243 (122.0875, 45.1) -> (121.5875, 44.6) centre (122.0875, 44.6) ccw
  line L252 (111.275, 31.1) -> (98.275, 31.1)
  line L253 (111.275, 45.1) -> (98.275, 45.1)
  line L254 (111.775, 31.6) -> (111.775, 44.6)
  line L255 (97.775, 31.6) -> (97.775, 44.6)
  arc A244 (111.275, 31.1) -> (111.775, 31.6) centre (111.275, 31.6) ccw
  arc A245 (97.775, 31.6) -> (98.275, 31.1) centre (98.275, 31.6) ccw
  arc A246 (111.775, 44.6) -> (111.275, 45.1) centre (111.275, 44.6) ccw
  arc A247 (98.275, 45.1) -> (97.775, 44.6) centre (98.275, 44.6) ccw
  line L256 (87.4625, 31.1) -> (74.4625, 31.1)
  line L257 (87.4625, 45.1) -> (74.4625, 45.1)
  line L258 (87.9625, 31.6) -> (87.9625, 44.6)
  line L259 (73.9625, 31.6) -> (73.9625, 44.6)
  arc A248 (87.4625, 31.1) -> (87.9625, 31.6) centre (87.4625, 31.6) ccw
  arc A249 (73.9625, 31.6) -> (74.4625, 31.1) centre (74.4625, 31.6) ccw
  arc A250 (87.9625, 44.6) -> (87.4625, 45.1) centre (87.4625, 44.6) ccw
  arc A251 (74.4625, 45.1) -> (73.9625, 44.6) centre (74.4625, 44.6) ccw
  line L260 (6.5, 31.1) -> (-6.5, 31.1)
  line L261 (6.5, 45.1) -> (-6.5, 45.1)
  line L262 (7, 31.6) -> (7, 44.6)
  line L263 (-7, 31.6) -> (-7, 44.6)
  arc A252 (6.5, 31.1) -> (7, 31.6) centre (6.5, 31.6) ccw
  arc A253 (-7, 31.6) -> (-6.5, 31.1) centre (-6.5, 31.6) ccw
  arc A254 (7, 44.6) -> (6.5, 45.1) centre (6.5, 44.6) ccw
  arc A255 (-6.5, 45.1) -> (-7, 44.6) centre (-6.5, 44.6) ccw
  line L264 (60.15, 32.1) -> (54.15, 32.1)
  line L265 (60.65, 32.6) -> (60.65, 45.625)
  line L266 (53.65, 32.6) -> (53.65, 45.625)
  arc A256 (60.15, 32.1) -> (60.65, 32.6) centre (60.15, 32.6) ccw
  arc A257 (53.65, 32.6) -> (54.15, 32.1) centre (54.15, 32.6) ccw
  line L267 (-54.15, 32.1) -> (-60.15, 32.1)
  line L268 (-53.65, 32.6) -> (-53.65, 45.625)
  line L269 (-60.65, 32.6) -> (-60.65, 45.625)
  arc A258 (-54.15, 32.1) -> (-53.65, 32.6) centre (-54.15, 32.6) ccw
  arc A259 (-60.65, 32.6) -> (-60.15, 32.1) centre (-60.15, 32.6) ccw
  line L270 (44.6, 31.1) -> (31.6, 31.1)
  line L271 (44.6, 45.1) -> (31.6, 45.1)
  line L272 (45.1, 31.6) -> (45.1, 44.6)
  line L273 (31.1, 31.6) -> (31.1, 44.6)
  arc A260 (44.6, 31.1) -> (45.1, 31.6) centre (44.6, 31.6) ccw
  arc A261 (31.1, 31.6) -> (31.6, 31.1) centre (31.6, 31.6) ccw
  arc A262 (45.1, 44.6) -> (44.6, 45.1) centre (44.6, 44.6) ccw
  arc A263 (31.6, 45.1) -> (31.1, 44.6) centre (31.6, 44.6) ccw
  line L274 (60.15, 32.1) -> (54.15, 32.1)
  line L275 (60.65, 32.6) -> (60.65, 45.625)
  line L276 (53.65, 32.6) -> (53.65, 45.625)
  arc A264 (60.15, 32.1) -> (60.65, 32.6) centre (60.15, 32.6) ccw
  arc A265 (53.65, 32.6) -> (54.15, 32.1) centre (54.15, 32.6) ccw
  line L277 (22.05, 32.1) -> (16.05, 32.1)
  line L278 (22.55, 32.6) -> (22.55, 45.625)
  line L279 (15.55, 32.6) -> (15.55, 45.625)
  arc A266 (22.05, 32.1) -> (22.55, 32.6) centre (22.05, 32.6) ccw
  arc A267 (15.55, 32.6) -> (16.05, 32.1) centre (16.05, 32.6) ccw
  line L280 (6.5, 31.1) -> (-6.5, 31.1)
  line L281 (6.5, 45.1) -> (-6.5, 45.1)
  line L282 (7, 31.6) -> (7, 44.6)
  line L283 (-7, 31.6) -> (-7, 44.6)
  arc A268 (6.5, 31.1) -> (7, 31.6) centre (6.5, 31.6) ccw
  arc A269 (-7, 31.6) -> (-6.5, 31.1) centre (-6.5, 31.6) ccw
  arc A270 (7, 44.6) -> (6.5, 45.1) centre (6.5, 44.6) ccw
  arc A271 (-6.5, 45.1) -> (-7, 44.6) centre (-6.5, 44.6) ccw
  line L284 (-31.6, 31.1) -> (-44.6, 31.1)
  line L285 (-31.6, 45.1) -> (-44.6, 45.1)
  line L286 (-31.1, 31.6) -> (-31.1, 44.6)
  line L287 (-45.1, 31.6) -> (-45.1, 44.6)
  arc A272 (-31.6, 31.1) -> (-31.1, 31.6) centre (-31.6, 31.6) ccw
  arc A273 (-45.1, 31.6) -> (-44.6, 31.1) centre (-44.6, 31.6) ccw
  arc A274 (-31.1, 44.6) -> (-31.6, 45.1) centre (-31.6, 44.6) ccw
  arc A275 (-44.6, 45.1) -> (-45.1, 44.6) centre (-44.6, 44.6) ccw
  line L288 (-16.05, 32.1) -> (-22.05, 32.1)
  line L289 (-15.55, 32.6) -> (-15.55, 45.625)
  line L290 (-22.55, 32.6) -> (-22.55, 45.625)
  arc A276 (-16.05, 32.1) -> (-15.55, 32.6) centre (-16.05, 32.6) ccw
  arc A277 (-22.55, 32.6) -> (-22.05, 32.1) centre (-22.05, 32.6) ccw
  line L291 (-54.15, 32.1) -> (-60.15, 32.1)
  line L292 (-53.65, 32.6) -> (-53.65, 45.625)
  line L293 (-60.65, 32.6) -> (-60.65, 45.625)
  arc A278 (-54.15, 32.1) -> (-53.65, 32.6) centre (-54.15, 32.6) ccw
  arc A279 (-60.65, 32.6) -> (-60.15, 32.1) centre (-60.15, 32.6) ccw
  line L294 (-74.4625, 31.1) -> (-87.4625, 31.1)
  line L295 (-74.4625, 45.1) -> (-87.4625, 45.1)
  line L296 (-73.9625, 31.6) -> (-73.9625, 44.6)
  line L297 (-87.9625, 31.6) -> (-87.9625, 44.6)
  arc A280 (-74.4625, 31.1) -> (-73.9625, 31.6) centre (-74.4625, 31.6) ccw
  arc A281 (-87.9625, 31.6) -> (-87.4625, 31.1) centre (-87.4625, 31.6) ccw
  arc A282 (-73.9625, 44.6) -> (-74.4625, 45.1) centre (-74.4625, 44.6) ccw
  arc A283 (-87.4625, 45.1) -> (-87.9625, 44.6) centre (-87.4625, 44.6) ccw
  line L298 (-98.275, 31.1) -> (-111.275, 31.1)
  line L299 (-98.275, 45.1) -> (-111.275, 45.1)
  line L300 (-97.775, 31.6) -> (-97.775, 44.6)
  line L301 (-111.775, 31.6) -> (-111.775, 44.6)
  arc A284 (-98.275, 31.1) -> (-97.775, 31.6) centre (-98.275, 31.6) ccw
  arc A285 (-111.775, 31.6) -> (-111.275, 31.1) centre (-111.275, 31.6) ccw
  arc A286 (-97.775, 44.6) -> (-98.275, 45.1) centre (-98.275, 44.6) ccw
  arc A287 (-111.275, 45.1) -> (-111.775, 44.6) centre (-111.275, 44.6) ccw
  line L302 (-122.0875, 31.1) -> (-135.0875, 31.1)
  line L303 (-122.0875, 45.1) -> (-135.0875, 45.1)
  line L304 (-121.5875, 31.6) -> (-121.5875, 44.6)
  line L305 (-135.5875, 31.6) -> (-135.5875, 44.6)
  arc A288 (-122.0875, 31.1) -> (-121.5875, 31.6) centre (-122.0875, 31.6) ccw
  arc A289 (-135.5875, 31.6) -> (-135.0875, 31.1) centre (-135.0875, 31.6) ccw
  arc A290 (-121.5875, 44.6) -> (-122.0875, 45.1) centre (-122.0875, 44.6) ccw
  arc A291 (-135.0875, 45.1) -> (-135.5875, 44.6) centre (-135.0875, 44.6) ccw
  line L306 (140.875, -47.625) -> (-140.875, -47.625)
  line L307 (142.875, 45.625) -> (142.875, -45.625)
  line L308 (-142.875, 45.625) -> (-142.875, -45.625)
  line L309 (-107.8, -31.1) -> (-107.887, -31.1)
  line L310 (-115.887, -31.1) -> (-120.8, -31.1)
  line L311 (-126.85, -31.1) -> (-131.763, -31.1)
  line L312 (-139.763, -31.1) -> (-139.85, -31.1)
  line L313 (-100.6563, 26.05) -> (-100.7432, 26.05)
  line L314 (-108.7433, 26.05) -> (-113.6563, 26.05)
  line L315 (140.875, 47.625) -> (62.65, 47.625)
  line L316 (51.65, 47.625) -> (24.55, 47.625)
  line L317 (13.55, 47.625) -> (-13.55, 47.625)
  line L318 (-24.55, 47.625) -> (-51.65, 47.625)
  line L319 (-62.65, 47.625) -> (-140.875, 47.625)
  arc A292 (142.875, 45.625) -> (140.875, 47.625) centre (140.875, 45.625) ccw
  arc A293 (62.65, 47.625) -> (60.65, 45.625) centre (62.65, 45.625) ccw
  arc A294 (53.65, 45.625) -> (51.65, 47.625) centre (51.65, 45.625) ccw
  arc A295 (24.55, 47.625) -> (22.55, 45.625) centre (24.55, 45.625) ccw
  arc A296 (15.55, 45.625) -> (13.55, 47.625) centre (13.55, 45.625) ccw
  arc A297 (-13.55, 47.625) -> (-15.55, 45.625) centre (-13.55, 45.625) ccw
  arc A298 (-22.55, 45.625) -> (-24.55, 47.625) centre (-24.55, 45.625) ccw
  arc A299 (-51.65, 47.625) -> (-53.65, 45.625) centre (-51.65, 45.625) ccw
  arc A300 (-60.65, 45.625) -> (-62.65, 47.625) centre (-62.65, 45.625) ccw
  arc A301 (140.875, -47.625) -> (142.875, -45.625) centre (140.875, -45.625) ccw
  arc A302 (-142.875, -45.625) -> (-140.875, -47.625) centre (-140.875, -45.625) ccw
  arc A303 (-140.875, 47.625) -> (-142.875, 45.625) centre (-140.875, 45.625) ccw
  arc A304 (-101.2432, 26.55) -> (-100.7432, 26.05) centre (-100.7432, 26.55) ccw
  arc A305 (-108.7433, 26.05) -> (-108.2433, 26.55) centre (-108.7433, 26.55) ccw
  arc A306 (-132.6193, 26.05) -> (-132.1193, 26.55) centre (-132.6193, 26.55) ccw
  arc A307 (-125.85, 13.05) -> (-126.35, 12.55) centre (-125.85, 12.55) ccw
  arc A308 (-108.387, -30.6) -> (-107.887, -31.1) centre (-107.887, -30.6) ccw
  arc A309 (-115.887, -31.1) -> (-115.387, -30.6) centre (-115.887, -30.6) ccw
  arc A310 (-132.263, -30.6) -> (-131.763, -31.1) centre (-131.763, -30.6) ccw
  arc A311 (-139.763, -31.1) -> (-139.263, -30.6) centre (-139.763, -30.6) ccw
  point P0 (0, 0)
  dimension "d0" = 2
  dimension "d1" = 2
  dimension "d2" = 2
  dimension "d3" = 2
  dimension "d4" = 2
  dimension "d5" = 2
  dimension "d6" = 0.5
  constraints: 640 end point, 624 point on circle, 312 centre point, 38 tangent, 13 equal radius, 12 point on line
  measures "d0" radius of A292
  measures "d1" radius of A293
  measures "d2" radius of A294
  measures "d3" radius of A295
  measures "d4" radius of A297
  measures "d5" radius of A301
  measures "d6" radius of A304
extrude "Extrusion1" add sketch "Sketch1" along normal blind 1.5
sketch "Sketch2" plane through (0, 0, 0) normal (0, -1, 0) x (1, 0, 0)
  point P0 (0, 0)
sketch "Sketch4" plane through (0, 1.5, 0) normal (0, 1, 0) x (1, 0, 0)
  line L0 (-141.35, 48.1) -> (141.35, 48.1)
  line L1 (143.35, 46.1) -> (143.35, -27.05)
  line L2 (93.725, -48.1) -> (-93.725, -48.1)
  line L3 (-143.35, -27.05) -> (-143.35, 46.1)
  line L4 (-139.85, 45.1) -> (-126.85, 45.1) projected
  line L5 (-140.35, 31.6) -> (-140.35, 44.6) projected
  line L6 (-122.0875, -45.1) -> (-135.0875, -45.1) projected
  line L7 (140.35, 44.6) -> (140.35, 31.6) projected
  line L8 (-141.35, -29.05) -> (-96.725, -29.05)
  line L9 (-95.725, -30.05) -> (-95.725, -46.1)
  line L10 (-114.9437, -26.05) -> (-127.9437, -26.05) projected
  line L11 (-97.775, -31.6) -> (-97.775, -44.6) projected
  line L12 (141.35, -29.05) -> (96.725, -29.05)
  line L13 (95.725, -30.05) -> (95.725, -46.1)
  line L14 (97.775, -44.6) -> (97.775, -31.6) projected
  line L15 (123.1813, -26.05) -> (108.7433, -26.05) projected
  line L16 (-144.35, -54.1) -> (144.35, -54.1)
  line L17 (146.35, -52.1) -> (146.35, 52.1)
  line L18 (144.35, 54.1) -> (-144.35, 54.1)
  line L19 (-146.35, 52.1) -> (-146.35, -52.1)
  arc A0 (-141.35, 48.1) -> (-143.35, 46.1) centre (-141.35, 46.1) ccw
  arc A1 (-143.35, -27.05) -> (-141.35, -29.05) centre (-141.35, -27.05) ccw
  arc A2 (-95.725, -46.1) -> (-93.725, -48.1) centre (-93.725, -46.1) ccw
  arc A3 (141.35, -29.05) -> (143.35, -27.05) centre (141.35, -27.05) ccw
  arc A4 (93.725, -48.1) -> (95.725, -46.1) centre (93.725, -46.1) ccw
  arc A5 (-95.725, -30.05) -> (-96.725, -29.05) centre (-96.725, -30.05) ccw
  arc A6 (96.725, -29.05) -> (95.725, -30.05) centre (96.725, -30.05) ccw
  arc A7 (143.35, 46.1) -> (141.35, 48.1) centre (141.35, 46.1) ccw
  arc A8 (-144.35, 54.1) -> (-146.35, 52.1) centre (-144.35, 52.1) ccw
  arc A9 (-146.35, -52.1) -> (-144.35, -54.1) centre (-144.35, -52.1) ccw
  arc A10 (144.35, -54.1) -> (146.35, -52.1) centre (144.35, -52.1) ccw
  arc A11 (146.35, 52.1) -> (144.35, 54.1) centre (144.35, 52.1) ccw
  point P0 (0, 0)
  dimension "d9" = 3
  dimension "d10" = 3
  dimension "d11" = 3
  dimension "d12" = 3
  dimension "d13" = 3
  dimension "d14" = 2.05
  dimension "d15" = 2.05
  dimension "d16" = 3
  dimension "d17" = 3
  dimension "d18" = 3
  dimension "d19" = 6
  dimension "d20" = 6
  dimension "d21" = 2
  dimension "d22" = 1
  dimension "d23" = 2
  constraints: 24 end point, 24 point on circle, 24 tangent, 12 centre point, 9 equal radius, 8 perpendicular, 4 horizontal
  measures "d9" distance between parallel lines of L4 L0
  measures "d10" distance between parallel lines of L5 L3
  measures "d11" distance between parallel lines of L2 L6
  measures "d12" distance between parallel lines of L1 L7
  measures "d13" distance between parallel lines of L8 L10
  measures "d14" distance between parallel lines of L9 L11
  measures "d15" distance between parallel lines of L13 L14
  measures "d16" distance between parallel lines of L15 L12
  measures "d17" distance between parallel lines of L3 L19
  measures "d18" distance between parallel lines of L17 L1
  measures "d19" distance between parallel lines of L0 L18
  measures "d20" distance between parallel lines of L16 L2
  measures "d21" radius of A0
  measures "d22" radius of A5
  measures "d23" radius of A7
body "Solid1"
